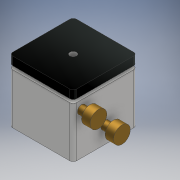
# Autodesk Inventor part: RadiantDyes-RD-PDT-S(appox)
Saved by Autodesk Inventor 2017 (Build 210142000, 142)
## iProperties
Created: 2022-03-01
Part Number: RadiantDyes-RD-PDT-S(appox)
Material: Generic
Document SubType Name: Modeling
Designer: Nikita
Density: 1 g/cm^3
Appearance: Default
Author: Nikita
Autodesk Inventor part; units mm, degrees
ref_plane "YZ Plane" through (0, 0, 0) normal (1, 0, 0) x (0, 1, 0)
ref_plane "XZ Plane" through (0, 0, 0) normal (0, 1, 0) x (-1, 0, 0)
ref_plane "XY Plane" through (0, 0, 0) normal (0, 0, 1) x (1, 0, 0)
sketch "Sketch1" plane through (0, 0, 0) normal (0, 0, 1) x (1, 0, 0)
  line L0 (19, -19) -> (-19, -19)
  line L1 (-19, -19) -> (-19, 19)
  line L2 (-19, 19) -> (19, 19)
  line L3 (19, 19) -> (19, -19)
  line L4 (19, -19) -> (-19, 19) construction
  line L5 (-19, -19) -> (19, 19) construction
  point P0 (0, 0)
  dimension "d0" = 38
  dimension "d1" = 38
  constraints: 12 end point, 2 midpoint, 2 parallel, 1 horizontal, 1 perpendicular
  measures "d0" distance of L1.end L2.end
  measures "d1" distance of L0.end L1.end
extrude "Extrusion1" add sketch "Sketch1" along normal blind 30
sketch "Sketch2" plane through (0, 0, 30) normal (0, 0, 1) x (1, 0, 0)
  circle A0 centre (0, 0) radius 2.5
  dimension "d4" = 5
  constraints: 1 centre point, 1 coincident
  measures "d4" diameter of A0
extrude "Extrusion2" add sketch "Sketch2" along normal blind 2
sketch "Sketch3" plane through (0, 0, 32) normal (0, 0, 1) x (1, 0, 0)
  line L0 (19, 19) -> (-19, 19) projected
  line L1 (-19, 19) -> (-19, -19) projected
  line L2 (-19, -19) -> (19, -19) projected
  line L3 (19, -19) -> (19, 19) projected
  point P0 (0, 0)
extrude "Extrusion3" add sketch "Sketch3" along normal blind 5
sketch "Sketch4" plane through (-19, 19, 0) normal (0, 1, 0) x (1, 0, 0)
  circle A0 centre (19, -10) radius 2.5
  point P0 (19, 0)
  dimension "d9" = 5
  constraints: 1 centre point
  measures "d9" diameter of A0
extrude "Extrusion4" add sketch "Sketch4" along normal blind 5
sketch "Sketch5" plane through (0, 24, 10) normal (0, 1, 0) x (1, 0, 0)
  circle A0 centre (0, 0) radius 5
  point P0 (0, 10)
  dimension "d12" = 10
  constraints: 1 centre point
  measures "d12" diameter of A0
extrude "Extrusion5" add sketch "Sketch5" along normal blind 5
sketch "Sketch6" plane through (19, -19, 0) normal (1, 0, 0) x (0, 0, -1)
  circle A0 centre (-10, 19) radius 2.5
  circle A1 centre (-25, 5) radius 2.5
  point P0 (0, 19)
  dimension "d15" = 5
  dimension "d16" = 5
  constraints: 2 centre point
  measures "d15" diameter of A0
  measures "d16" diameter of A1
extrude "Extrusion6" add sketch "Sketch6" along normal blind 5
sketch "Sketch7" plane through (24, 0, 10) normal (1, 0, 0) x (0, 0, -1)
  circle A0 centre (0, 0) radius 5
  circle A1 centre (-15, -14) radius 2.5 projected
  circle A2 centre (-15, -14) radius 5
  point P0 (10, 0)
  dimension "d19" = 10
  dimension "d20" = 10
  constraints: 2 centre point, 1 coincident
  measures "d19" diameter of A0
  measures "d20" diameter of A2
extrude "Extrusion7" add sketch "Sketch7" along normal blind 5 contours A0 | A1 | A2
fillet "Fillet1" radius 2 8 edges at (19, 19, 15) (19, 19, 34.5) (19, -19, 15) (-19, 19, 15) (19, -19, 34.5) (-19, -19, 15) (-19, -19, 34.5) (-19, 19, 34.5)
sketch "Sketch8" plane through (0, 0, 37) normal (0, 0, 1) x (1, 0, 0)
  circle A0 centre (0, 0) radius 2
  dimension "d24" = 4
  constraints: 1 centre point, 1 coincident
  measures "d24" diameter of A0
extrude "Extrusion8" cut sketch "Sketch8" against normal blind 5
body "Solid1"
